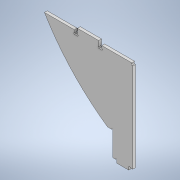
# Autodesk Inventor part: Support A1 - V2
Saved by Autodesk Inventor 2020 (Build 240168000, 168)
## iProperties
Created: 2020-07-22
Part Number: Support A1 - V2
Material: Generic
Document SubType Name: Modeling
Designer: Dan Wikman
Density: 1 g/cm^3
Appearance: Default
Author: Dan Wikman
Autodesk Inventor part; units mm, degrees
ref_plane "YZ Plane" through (0, 0, 0) normal (1, 0, 0) x (0, 1, 0)
ref_plane "XZ Plane" through (0, 0, 0) normal (0, 1, 0) x (-1, 0, 0)
ref_plane "XY Plane" through (0, 0, 0) normal (0, 0, 1) x (1, 0, 0)
sketch "Sketch1" plane through (0, 0, 0) normal (0, 0, 1) x (1, 0, 0)
  arc A0 (0, 550) -> (-200, 512.3475) centre (0, 0) ccw construction
  line L0 (-472.3938, -281.6809) -> (-252.3938, -281.6809) construction
  line L1 (-489.0365, 251.6809) -> (-252.3938, 251.6809) construction
  line L2 (-150, 323.3356) -> (-150, 512.3475) construction
  line L3 (-472.3938, 281.6809) -> (-252.3938, 281.6809) construction
  line L4 (-472.3938, -251.6809) -> (-252.3938, -251.6809) construction
  line L5 (-356.435, 15) -> (-576.435, 15) construction
  line L6 (-472.3938, -281.6809) -> (-472.3938, -251.6809) construction
  line L7 (-252.3938, -281.6809) -> (-252.3938, -251.6809) construction
  line L8 (-252.3938, 281.6809) -> (-252.3938, 251.6809) construction
  line L9 (-472.3938, 281.6809) -> (-472.3938, 251.6809) construction
  line L10 (-356.435, 15) -> (-356.435, -15) construction
  line L11 (-356.435, -15) -> (-576.435, -15) construction
  line L12 (-576.435, -15) -> (-576.435, 15) construction
  arc A1 (0, 356.435) -> (-150, 323.3356) centre (0, 0) ccw construction
  arc A2 (-150, -323.3356) -> (0, -356.435) centre (0, 0) ccw construction
  arc A3 (-256.5, -512.3475) -> (-260, -512.3475) centre (-258.25, -512.3475) ccw
  arc A4 (-290, -512.3475) -> (-293.5, -512.3475) centre (-291.75, -512.3475) ccw
  line L13 (-356.1192, -15) -> (-549.7954, -15) construction
  line L14 (-252.3938, 251.6809) -> (-489.0365, 251.6809) construction
  arc A5 (-192.6667, 512.3475) -> (-190, 512.3475) centre (-191.3333, 512.3475) ccw construction
  line L15 (-157.3333, 512.3475) -> (-150, 512.3475) construction
  line L16 (-192.6667, 512.3475) -> (-200, 512.3475) construction
  arc A6 (-160, 512.3475) -> (-157.3333, 512.3475) centre (-158.6667, 512.3475) ccw construction
  line L17 (-171.25, 517.8475) -> (-175, 517.8475) construction
  line L18 (-171.25, 520.5142) -> (-171.25, 525.1809) construction
  line L19 (-161.3333, 532.3475) -> (-188.6667, 532.3475) construction
  line L20 (-190, 531.0142) -> (-190, 512.3475) construction
  line L21 (-160, 531.0142) -> (-160, 512.3475) construction
  arc A7 (-160, 531.0142) -> (-161.3333, 532.3475) centre (-161.3333, 531.0142) ccw construction
  arc A8 (-188.6667, 532.3475) -> (-190, 531.0142) centre (-188.6667, 531.0142) ccw construction
  line L22 (-171.25, 527.8475) -> (-175, 527.8475) construction
  line L23 (-175, 532.3475) -> (-175, 535.9358) construction
  line L24 (-175, 517.8475) -> (-175, 527.8475) construction
  arc A9 (-171.25, 517.8475) -> (-171.25, 520.5142) centre (-171.25, 519.1809) ccw construction
  arc A10 (-171.25, 525.1809) -> (-171.25, 527.8475) centre (-171.25, 526.5142) ccw construction
  line L25 (-178.75, 517.8475) -> (-175, 517.8475) construction
  arc A11 (-178.75, 520.5142) -> (-178.75, 517.8475) centre (-178.75, 519.1809) ccw construction
  line L26 (-178.75, 520.5142) -> (-178.75, 525.1809) construction
  arc A12 (-178.75, 527.8475) -> (-178.75, 525.1809) centre (-178.75, 526.5142) ccw construction
  line L27 (-178.75, 527.8475) -> (-175, 527.8475) construction
  line L28 (-362.3938, -251.6809) -> (-362.3938, -293.6041)
  arc A13 (-389.2055, -291.6809) -> (-389.2055, -288.1809) centre (-389.2055, -289.9309) ccw
  line L29 (-389.2055, -291.6809) -> (-396.7055, -291.6809)
  line L30 (-396.7055, -281.6809) -> (-472.3938, -281.6809)
  line L31 (-328.082, -281.6809) -> (-252.3938, -281.6809)
  line L32 (-252.3938, -287.3475) -> (-250, -287.3475)
  arc A14 (-150, 323.3356) -> (-252.3938, -251.6809) centre (0, 0) ccw construction
  arc A15 (-200, 512.3475) -> (-472.3938, -281.6809) centre (0, 0) ccw construction
  line L33 (-300, -512.3475) -> (-300, -491.6809)
  line L34 (-260, -512.3475) -> (-260, -519.3475)
  line L35 (-290, -519.3475) -> (-290, -512.3475)
  line L36 (-256.5, -512.3475) -> (-250, -512.3475)
  line L37 (-293.5, -512.3475) -> (-300, -512.3475)
  arc A16 (-396.7055, -288.1809) -> (-396.7055, -291.6809) centre (-396.7055, -289.9309) ccw
  line L38 (-396.7055, -281.6809) -> (-396.7055, -288.1809)
  line L39 (-389.2055, -288.1809) -> (-389.2055, -274.6809)
  arc A17 (-335.582, -288.1809) -> (-335.582, -291.6809) centre (-335.582, -289.9309) ccw
  line L40 (-335.582, -291.6809) -> (-328.082, -291.6809)
  arc A18 (-328.082, -291.6809) -> (-328.082, -288.1809) centre (-328.082, -289.9309) ccw
  line L41 (-328.082, -281.6809) -> (-328.082, -288.1809)
  line L42 (-335.582, -288.1809) -> (-335.582, -274.6809)
  arc A19 (-252.3938, -283.8475) -> (-252.3938, -287.3475) centre (-252.3938, -285.5975) ccw
  line L43 (-252.3938, -283.8475) -> (-252.3938, -281.6809)
  line L44 (-335.582, -274.6809) -> (-389.2055, -274.6809)
  arc A20 (-472.3938, -281.6809) -> (-313.5, -451.9046) centre (0, 0) ccw
  line L45 (-250, -512.3475) -> (-250, -287.3475)
  line L46 (-300, -491.6809) -> (-300, -451.9046)
  arc A21 (-300, -451.9046) -> (-303.5, -451.9046) centre (-301.75, -451.9046) ccw
  line L47 (-313.5, -451.9046) -> (-303.5, -451.9046)
  line L48 (-290, -519.3475) -> (-260, -519.3475)
  point P0 (0, 512.3475)
  point P1 (0, -512.3475)
  point P2 (-59.9119, -534.1417)
  point P3 (-160, 532.3475)
  point P4 (-190, 532.3475)
  point P5 (-335.582, -268.123)
  point P6 (-389.2055, -268.123)
  dimension "d13" = 550
  dimension "d17" = 200
  dimension "d18" = 0
  dimension "d54" = 220
  dimension "d56" = 220
  dimension "d57" = 30
  dimension "d59" = 30
  dimension "d62" = 252.3938
  dimension "d73" = 236.6809
  dimension "d74" = 236.6809
  dimension "d75" = 576.435
  dimension "d76" = 472.3938
  dimension "d77" = 472.3938
  dimension "d78" = 30
  dimension "d81" = 220
  dimension "d82" = 252.3938
  dimension "d85" = 356.435
  dimension "d88" = 3.5
  dimension "d91" = 3.5
  dimension "d105" = 2.6667
  dimension "d106" = 30
  dimension "d107" = 20
  dimension "d108" = 2.6667
  dimension "d109" = 1.3333
  dimension "d110" = 7.3333
  dimension "d111" = 7.3333
  dimension "d112" = 7.5
  dimension "d113" = 3.75
  dimension "d114" = 3.75
  dimension "d140" = 7.5
  dimension "d171" = 1.75
  dimension "d172" = 10
  dimension "d173" = 3.5
  dimension "d176" = 7
  dimension "d179" = 230.6667
  dimension "d182" = 3.5
  dimension "d183" = 7
  constraints: 98 end point, 49 point on circle, 22 centre point, 14 symmetric about line, 11 horizontal, 9 perpendicular, 6 vertical, 5 point on line, 2 collinear, 1 coincident, 1 midpoint, 1 parallel, 1 tangent, 4 other
  measures "d13" radius of A0
  measures "d17" distance of point (0, 512.348) A0.end
  measures "d18" horizontal distance of point (0, 0) point (0, 512.348)
  measures "d54" distance of L5.start L5.end
  measures "d56" distance of L0.start L0.end
  measures "d57" distance of L0.end L4.end
  measures "d59" distance between parallel lines of L3 L1
  measures "d62" distance from line of point (0, 0) L7
  measures "d73" distance between parallel lines of L4 L11
  measures "d74" distance between parallel lines of L1 L5
  measures "d75" distance from line of L12 point (0, 0)
  measures "d76" distance from line of point (0, 0) L6
  measures "d77" distance from line of point (0, 0) L9
  measures "d78" distance of L5.start L10.end
  measures "d81" distance between parallel lines of L8 L9
  measures "d82" distance from line of point (0, 0) L8
  measures "d85" distance from line of A0.centre L10
  measures "d88" diameter of A3
  measures "d91" diameter of A4
  measures "d105" diameter of A5
  measures "d106" distance of point (-160, 532.348) point (-190, 532.348)
  measures "d107" distance of point (-190, 532.348) L20.end
  measures "d108" diameter of A6
  measures "d109" radius of A7
  measures "d110" distance of L15.start L15.end
  measures "d111" distance of L16.start L16.end
  measures "d112" diameter of L18 L24
  measures "d113" distance of L17.start L17.end
  measures "d114" distance of L22.start L22.end
  measures "d140" distance of L29.start L29.end
  measures "d171" radius of A13
  measures "d172" distance between parallel lines of L30 L29
  measures "d173" diameter of A19
  measures "d176" distance between parallel lines of L0 L44
  measures "d179" distance between parallel lines of L0 L36
  measures "d182" diameter of A21
  measures "d183" distance between parallel lines of L36 L48
extrude "Extrusion1" add sketch "Sketch1" along normal blind 7
body "Solid1"
